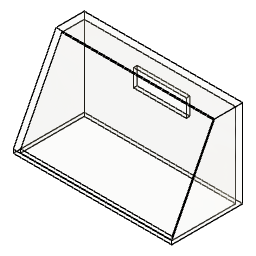
unsorted_smarties_holder (Autodesk Fusion 360 design; units mm, degrees)
Autodesk Fusion 360 part; units mm, degrees
sketch "Unsorted Smarties Holder" plane through (0, 0, 0) normal (1, 0, 0) x (0, 1, 0)
  line L0 (0, 0) -> (93.3717, 0)
  line L1 (93.3717, 0) -> (93.3717, 143.115)
  line L2 (93.3717, 143.115) -> (45.2924, 143.115)
  line L3 (45.2924, 143.115) -> (-27.6283, 0)
  line L4 (-27.6283, 0) -> (0, 0)
  line L5 (-27.6283, 0) -> (93.3717, 0)
  line L6 (93.3717, 0) -> (93.3717, -6)
  line L7 (93.3717, -6) -> (-27.6283, -6)
  line L8 (-27.6283, -6) -> (-27.6283, 0)
  dimension "d5" = 143.115
  dimension "d14" = 63
  dimension "d23" = 121
  dimension "d31" = 6
  constraint horizontal L0
  constraint vertical L1
  constraint horizontal L2
  constraint coincident L0.start L4.end
  constraint horizontal L5
  constraint vertical L6
  constraint horizontal L7
  constraint vertical L8
  constraint collinear L1 L6
  measures "d5" distance of L0.end L1.end
  measures "d14" angle of L3 L4
  measures "d23" distance of L0.end L3.end
  measures "d31" distance of L0 L7
extrude "Extrude1" add sketch "Unsorted Smarties Holder" along normal blind 270
sketch "Sketch3" plane through (270, 0, 0) normal (1, 0, 0) x (0, 1, 0)
  line L0 (93.3717, -6) -> (93.3717, 143.115)
  line L1 (93.3717, 143.115) -> (45.2924, 143.115)
  line L2 (45.2924, 143.115) -> (-27.6283, 0)
  line L3 (87.3717, 137.115) -> (87.3717, 0)
  line L4 (87.3717, 0) -> (-20.8944, 0)
  line L5 (-20.8944, 0) -> (48.9692, 137.115)
  line L6 (48.9692, 137.115) -> (87.3717, 137.115)
  line L7 (-27.6283, 0) -> (-27.6283, -6)
  line L8 (-27.6283, -6) -> (93.3717, -6)
  line L9 (-20.8944, 0) -> (87.3717, 0)
  line L10 (87.3717, 0) -> (87.3717, -6)
  line L11 (87.3717, -6) -> (-20.8944, -6)
  line L12 (-20.8944, -6) -> (-20.8944, 0)
  dimension "d15" = 6
  dimension "d16" = 6
  dimension "d17" = 6
  dimension "d18" = 6
  dimension "d32" = 6
  dimension "d33" = 6
  constraint perpendicular L1 L3
  constraint perpendicular L3 L4
  constraint parallel L2 L5
  constraint horizontal L9
  constraint vertical L10
  constraint horizontal L11
  constraint vertical L12
  constraint coincident L8 L10.end
  constraint collinear L3 L10
  measures "d15" distance of L1 L5.end
  measures "d16" distance of L1 L3.start
  measures "d17" distance of L2 L5
  measures "d18" distance of L0 L3
  measures "d32" distance of L4 L8
  measures "d33" distance of L9 L11
extrude "Extrude3" cut sketch "Sketch3" against normal blind 258 from surface at -6 contours L4 L8 L9 L10 L11 L12 | L3 L4 L5 L6 L9
sketch "Smarties Feed" plane through (0, 93.3717, 0) normal (0, 1, 0) x (-1, 0, 0)
  line L0 (0, -6) -> (0, 143.115)
  line L1 (0, 143.115) -> (-270, 143.115)
  line L2 (-270, 143.115) -> (-270, -6)
  line L3 (-180, 108.115) -> (-90, 108.115)
  line L4 (-90, 108.115) -> (-90, 78.115)
  line L5 (-90, 78.115) -> (-180, 78.115)
  line L6 (-180, 78.115) -> (-180, 108.115)
  line L7 (-270, -6) -> (0, -6)
  dimension "d24" = 30
  dimension "d25" = 90
  dimension "d26" = 90
  dimension "d27" = 90
  dimension "d28" = 35
  constraint horizontal L3
  constraint vertical L4
  constraint horizontal L5
  constraint vertical L6
  measures "d24" distance of L3.end L4.end
  measures "d25" distance of L3.start L3.end
  measures "d26" distance of L2 L6
  measures "d27" distance of L0 L4
  measures "d28" distance of L1 L3
extrude "Extrude4" cut sketch "Smarties Feed" against normal blind 6 contours L3 L4 L5 L6
equation "polycarbonateThickness = 6 mm" comment "Thickness of the polycarbonate panels"
equation "d14 = 180 deg - 117 deg"
equation "d15 = polycarbonateThickness"
equation "d16 = polycarbonateThickness"
equation "d17 = polycarbonateThickness"
equation "d18 = polycarbonateThickness"
equation "d20 = -polycarbonateThickness"
equation "d21 = -( 270 mm - 2 * polycarbonateThickness )"
equation "d28 = 41 mm - 6 mm"
equation "d29 = -polycarbonateThickness"
named bodies: "Unsorted Smarties Holder"
